Autodesk Fusion 360 part; units mm, degrees
note: some values were not read from the file. Chosen so that the rebuilt part matches the saved one: which face or edge a step refers to. Set by a fixed rule: which sketch regions a step uses.
(part 2 of 2)
sketch "Sketch18" plane through (0, 5, 0) normal (0, 1, 0) x (-1, 0, 0)
  line L0 (114.8227, 27.0674) -> (114.8227, -2.7993)
  line L1 (114.8227, -2.7993) -> (107.5823, -2.7993)
  line L2 (107.5823, -2.7993) -> (107.5823, 27.0674)
  line L3 (107.5823, 27.0674) -> (114.8227, 27.0674)
  line L4 (58, -24) -> (58, -27)
  line L5 (58, -27) -> (18, -27)
  line L6 (18, -27) -> (18, -24)
  line L7 (18, -24) -> (58, -24)
  line L8 (-10.8736, -33.1025) -> (-10.8736, -37.1025)
  line L9 (-10.8736, -37.1025) -> (-40.8736, -37.1025)
  line L10 (-40.8736, -37.1025) -> (-40.8736, -33.1025)
  line L11 (-40.8736, -33.1025) -> (-10.8736, -33.1025)
  circle A0 centre (-6.976, 41.8165) radius 1.5
  line L12 (-78.4638, 67.7606) -> (-78.4638, 30)
  line L13 (-78.4638, 30) -> (-84.4638, 30)
  line L14 (-84.4638, 30) -> (-84.4638, 67.7606)
  line L15 (-84.4638, 67.7606) -> (-78.4638, 67.7606)
  line L16 (-45, 85) -> (-45, 75)
  line L17 (-45, 75) -> (-85, 75)
  line L18 (-85, 75) -> (-85, 85)
  line L19 (-85, 85) -> (-45, 85)
  line L20 (-4.2145, 80) -> (-4.2145, 53.7294)
  line L21 (-4.2145, 53.7294) -> (-9.1198, 53.7294)
  line L22 (-9.1198, 53.7294) -> (-9.1198, 80)
  line L23 (-9.1198, 80) -> (-4.2145, 80)
  line L24 (-82.9645, 18.0619) -> (-82.9645, -13.0755)
  line L25 (-82.9645, -13.0755) -> (-89.1235, -13.0755)
  line L26 (-89.1235, -13.0755) -> (-89.1235, 18.0619)
  line L27 (-89.1235, 18.0619) -> (-82.9645, 18.0619)
  line L28 (44.7011, 105) -> (44.7011, 92.7786)
  line L29 (44.7011, 92.7786) -> (10, 92.7786)
  line L30 (10, 92.7786) -> (10, 105)
  line L31 (10, 105) -> (44.7011, 105)
  line L32 (-100, 38.7801) -> (-100, -17.7685)
  line L33 (-100, -17.7685) -> (-109.4869, -17.7685)
  line L34 (-109.4869, -17.7685) -> (-109.4869, 38.7801)
  line L35 (-109.4869, 38.7801) -> (-100, 38.7801)
  line L36 (0, 105) -> (0, 92.7786)
  line L37 (0, 92.7786) -> (-35, 92.7786)
  line L38 (-35, 92.7786) -> (-35, 105)
  line L39 (-35, 105) -> (0, 105)
  line L40 (-2.8969, 25.8787) -> (-2.8969, -24.0249)
  line L41 (-2.8969, -24.0249) -> (-8.0295, -24.0249)
  line L42 (-8.0295, -24.0249) -> (-8.0295, 25.8787)
  line L43 (-8.0295, 25.8787) -> (-2.8969, 25.8787)
  circle A1 centre (-97.7344, 53.0689) radius 5.2675
  circle A2 centre (97.7344, 53.0689) radius 5.2675
  circle A3 centre (92.5, -14.3) radius 1.6
  circle A4 centre (2.5, 75.7) radius 1.6
  circle A5 centre (92.5, 75.7) radius 1.6
  circle A6 centre (92.5, -17.7) radius 1.6
  circle A7 centre (92.5, -10.9) radius 1.6
  circle A8 centre (2.5, 72.3) radius 1.6
  circle A9 centre (92.5, 72.3) radius 1.6
  circle A10 centre (2.5, -14.3) radius 1.6
  circle A11 centre (-90.9905, 60.7002) radius 1.5
  circle A12 centre (90.8662, 44.7011) radius 1.5
  circle A13 centre (-90.8662, 44.7011) radius 1.5
  circle A14 centre (104.8647, 60.7002) radius 1.5
  circle A15 centre (90.9999, 67.3221) radius 1.5
  circle A16 centre (-104.8647, 60.7002) radius 1.5
  circle A17 centre (105.0292, 44.701) radius 1.5
  arc A18 (-105.0048, 43.2011) -> (-105.0133, 46.2009) centre (-104.989, 44.7011) ccw
  arc A19 (-105.0133, 46.2009) -> (-105.0048, 43.2011) centre (-105.0292, 44.701) ccw
  circle A20 centre (90.8944, 60.7176) radius 1.5
  circle A21 centre (0, -58) radius 2.45
  circle A22 centre (0, -116) radius 2.45
  circle A23 centre (104.95, 64) radius 1.5
  circle A24 centre (-90.95, 48) radius 1.5
  circle A25 centre (104.95, 48) radius 1.5
  circle A26 centre (-90.95, 64) radius 1.5
  circle A27 centre (-104.95, 64) radius 1.5
  circle A28 centre (90.95, 48) radius 1.5
  circle A29 centre (90.95, 64) radius 1.5
  circle A30 centre (-104.95, 48) radius 1.5
  line L44 (74, 33) -> (74, 28)
  line L45 (74, 28) -> (30, 28)
  line L46 (30, 28) -> (30, 33)
  line L47 (30, 33) -> (74, 33)
  line L48 (-30, 28) -> (-74, 28)
  line L49 (-74, 28) -> (-74, 33)
  line L50 (-74, 33) -> (-30, 33)
  line L51 (-30, 33) -> (-30, 28)
  line L52 (-112.5, 43.0811) -> (-117.3415, 43.0811)
  arc A31 (-117.3415, 43.0811) -> (117.3415, 43.0811) centre (0, 0) ccw
  line L53 (117.3415, 43.0811) -> (112.5, 43.0811)
  line L54 (112.5, 43.0811) -> (112.5, 68.0811)
  line L55 (112.5, 68.0811) -> (104.833, 68.0811)
  arc A32 (104.833, 68.0811) -> (-104.833, 68.0811) centre (0, 0) ccw
  line L56 (-104.833, 68.0811) -> (-112.5, 68.0811)
  line L57 (-112.5, 68.0811) -> (-112.5, 43.0811)
  circle A33 centre (91.5428, 79.2656) radius 1.6
  circle A34 centre (2.5, 79.1) radius 1.6
  circle A35 centre (-80.0985, -43.3755) radius 1.7
  circle A36 centre (20.0985, -43.3755) radius 1.7
  circle A37 centre (20.0985, -87.3755) radius 1.7
  circle A38 centre (-20.0985, -87.3755) radius 1.7
  circle A39 centre (-80.0985, -87.3755) radius 1.7
  circle A40 centre (80.0985, -43.3755) radius 1.7
  circle A41 centre (80.0985, -87.3755) radius 1.7
  circle A42 centre (-20.0985, -43.3755) radius 1.7
  line L58 (-85, -25) -> (-65.7302, -25)
  line L59 (-65.7302, -25) -> (-65.7302, -31)
  line L60 (-65.7302, -31) -> (-85, -31)
  line L61 (-85, -31) -> (-85, -25)
  line L62 (102.0125, -33.4763) -> (110, -33.4763)
  line L63 (110, -33.4763) -> (110, -40)
  line L64 (110, -40) -> (102.0125, -40)
  line L65 (102.0125, -40) -> (102.0125, -33.4763)
  dimension "d163" = 6
  constraint horizontal L58
  constraint vertical L59
  constraint horizontal L60
  constraint vertical L61
  constraint horizontal L62
  constraint vertical L63
  constraint horizontal L64
  constraint vertical L65
  measures "d163" distance of L58.start L60.end
extrude "Extrude30" cut sketch "Sketch18" against normal blind 5 contours L58 L59 L60 L61 | L62 L63 L64 L65 bodies 1
sketch "Sketch19" plane through (0, 0, 0) normal (0, -1, 0) x (1, 0, 0)
  circle A0 centre (20.0985, -43.3755) radius 1.7
  circle A1 centre (-80.0985, -87.3755) radius 1.7
  circle A2 centre (-80.0985, -43.3755) radius 1.7
  circle A3 centre (80.0985, -87.3755) radius 1.7
  circle A4 centre (20.0985, -87.3755) radius 1.7
  circle A5 centre (-20.0985, -87.3755) radius 1.7
  circle A6 centre (-20.0985, -43.3755) radius 1.7
  circle A7 centre (80.0985, -43.3755) radius 1.7
  circle A8 centre (-2.5, 79.1) radius 1.6
  circle A9 centre (-91.5428, 79.2656) radius 1.6
  line L0 (117.3415, 43.0811) -> (112.5, 43.0811)
  line L1 (112.5, 43.0811) -> (112.5, 68.0811)
  line L2 (112.5, 68.0811) -> (104.833, 68.0811)
  arc A10 (104.833, 68.0811) -> (-104.833, 68.0811) centre (0, 0) ccw
  line L3 (-104.833, 68.0811) -> (-112.5, 68.0811)
  line L4 (-112.5, 68.0811) -> (-112.5, 43.0811)
  line L5 (-112.5, 43.0811) -> (-117.3415, 43.0811)
  arc A11 (-117.3415, 43.0811) -> (-10, -124.5994) centre (0, 0) ccw
  line L6 (-10, -124.5994) -> (-10, -45)
  line L7 (-10, -45) -> (10, -45)
  line L8 (10, -45) -> (10, -124.5994)
  arc A12 (10, -124.5994) -> (117.3415, 43.0811) centre (0, 0) ccw
  line L9 (74, 28) -> (30, 28)
  line L10 (30, 28) -> (30, 33)
  line L11 (30, 33) -> (74, 33)
  line L12 (74, 33) -> (74, 28)
  line L13 (-74, 28) -> (-74, 33)
  line L14 (-74, 33) -> (-30, 33)
  line L15 (-30, 33) -> (-30, 28)
  line L16 (-30, 28) -> (-74, 28)
  circle A13 centre (104.95, 48) radius 1.5
  circle A14 centre (-90.95, 64) radius 1.5
  circle A15 centre (-90.95, 48) radius 1.5
  circle A16 centre (104.95, 64) radius 1.5
  circle A17 centre (90.95, 64) radius 1.5
  circle A18 centre (-104.95, 48) radius 1.5
  circle A19 centre (90.95, 48) radius 1.5
  circle A20 centre (-104.95, 64) radius 1.5
  circle A21 centre (-90.8944, 60.7176) radius 1.5
  arc A22 (105.0133, 46.2009) -> (105.0048, 43.2011) centre (104.989, 44.7011) ccw
  arc A23 (105.0048, 43.2011) -> (105.0133, 46.2009) centre (105.0292, 44.701) ccw
  circle A24 centre (-105.0292, 44.701) radius 1.5
  circle A25 centre (-90.9999, 67.3221) radius 1.5
  circle A26 centre (-104.8647, 60.7002) radius 1.5
  circle A27 centre (90.8662, 44.7011) radius 1.5
  circle A28 centre (-90.8662, 44.7011) radius 1.5
  circle A29 centre (-2.5, -14.3) radius 1.6
  circle A30 centre (-92.5, 72.3) radius 1.6
  circle A31 centre (-2.5, 72.3) radius 1.6
  circle A32 centre (-92.5, -10.9) radius 1.6
  circle A33 centre (-92.5, -17.7) radius 1.6
  circle A34 centre (-92.5, 75.7) radius 1.6
  circle A35 centre (-2.5, 75.7) radius 1.6
  circle A36 centre (-92.5, -14.3) radius 1.6
  circle A37 centre (-97.7344, 53.0689) radius 5.2675
  circle A38 centre (97.7344, 53.0689) radius 5.2675
  line L17 (2.8969, -24.0249) -> (2.8969, 25.8787)
  line L18 (2.8969, 25.8787) -> (8.0295, 25.8787)
  line L19 (8.0295, 25.8787) -> (8.0295, -24.0249)
  line L20 (8.0295, -24.0249) -> (2.8969, -24.0249)
  line L21 (0, 92.7786) -> (0, 105)
  line L22 (0, 105) -> (35, 105)
  line L23 (35, 105) -> (35, 92.7786)
  line L24 (35, 92.7786) -> (0, 92.7786)
  line L25 (100, -17.7685) -> (100, 38.7801)
  line L26 (100, 38.7801) -> (109.4869, 38.7801)
  line L27 (109.4869, 38.7801) -> (109.4869, -17.7685)
  line L28 (109.4869, -17.7685) -> (100, -17.7685)
  line L29 (-44.7011, 92.7786) -> (-44.7011, 105)
  line L30 (-44.7011, 105) -> (-10, 105)
  line L31 (-10, 105) -> (-10, 92.7786)
  line L32 (-10, 92.7786) -> (-44.7011, 92.7786)
  line L33 (82.9645, -13.0755) -> (82.9645, 18.0619)
  line L34 (82.9645, 18.0619) -> (89.1235, 18.0619)
  line L35 (89.1235, 18.0619) -> (89.1235, -13.0755)
  line L36 (89.1235, -13.0755) -> (82.9645, -13.0755)
  line L37 (4.2145, 53.7294) -> (4.2145, 80)
  line L38 (4.2145, 80) -> (9.1198, 80)
  line L39 (9.1198, 80) -> (9.1198, 53.7294)
  line L40 (9.1198, 53.7294) -> (4.2145, 53.7294)
  line L41 (45, 75) -> (45, 85)
  line L42 (45, 85) -> (85, 85)
  line L43 (85, 85) -> (85, 75)
  line L44 (85, 75) -> (45, 75)
  line L45 (78.4638, 30) -> (78.4638, 67.7606)
  line L46 (78.4638, 67.7606) -> (84.4638, 67.7606)
  line L47 (84.4638, 67.7606) -> (84.4638, 30)
  line L48 (84.4638, 30) -> (78.4638, 30)
  circle A39 centre (6.976, 41.8165) radius 1.5
  line L49 (-114.8227, -2.7993) -> (-114.8227, 27.0674)
  line L50 (-114.8227, 27.0674) -> (-107.5823, 27.0674)
  line L51 (-107.5823, 27.0674) -> (-107.5823, -2.7993)
  line L52 (-107.5823, -2.7993) -> (-114.8227, -2.7993)
  line L53 (65.7302, -31) -> (65.7302, -25)
  line L54 (65.7302, -25) -> (85, -25)
  line L55 (85, -25) -> (85, -31)
  line L56 (85, -31) -> (65.7302, -31)
  line L57 (-110, -40) -> (-110, -33.4763)
  line L58 (-110, -33.4763) -> (-102.0125, -33.4763)
  line L59 (-102.0125, -33.4763) -> (-102.0125, -40)
  line L60 (-102.0125, -40) -> (-110, -40)
  arc A40 (17, -122) -> (74.3564, -98.5123) centre (0.1514, 0.9191) ccw
  line L61 (0, -124) -> (0, -59) construction
  line L62 (74.3564, -98.5123) -> (75.9114, -99.3099)
  line L63 (17, -122) -> (17, -123.8386)
  arc A41 (90.5, -84.5) -> (122.1341, -18.16) centre (-0.7621, -0.2695) ccw
  line L64 (122.1341, -18.16) -> (123.6738, -18.16)
  line L65 (90.5, -84.5) -> (91.4094, -85.2603)
  arc A42 (76.2789, 96.4429) -> (6.6664, 123.005) centre (2.8431, 8.486) ccw
  line L66 (76.2789, 96.4429) -> (77.7474, 97.8792)
  line L67 (6.6664, 123.005) -> (6.6664, 124.8221)
  arc A43 (-6.6664, 123.005) -> (-76.2789, 96.4429) centre (-2.8431, 8.486) ccw
  line L68 (-76.2789, 96.4429) -> (-77.7474, 97.8792)
  line L69 (-6.6664, 123.005) -> (-6.6664, 124.8221)
  line L70 (-122.1341, -18.16) -> (-123.6738, -18.16)
  arc A44 (-122.1341, -18.16) -> (-90.5, -84.5) centre (0.7621, -0.2695) ccw
  line L71 (-90.5, -84.5) -> (-91.4094, -85.2603)
  line L72 (-74.3564, -98.5123) -> (-75.9114, -99.3099)
  arc A45 (-74.3564, -98.5123) -> (-17, -122) centre (-0.1514, 0.9191) ccw
  line L73 (-17, -122) -> (-17, -123.8386)
  line L74 (55, -105) -> (35, -105)
  line L75 (35, -105) -> (35, -100)
  line L76 (35, -100) -> (55, -100)
  line L77 (55, -100) -> (55, -105)
  line L78 (-55, -100) -> (-55, -105)
  line L79 (-55, -105) -> (-35, -105)
  line L80 (-35, -100) -> (-55, -100)
  line L81 (-35, -105) -> (-35, -100)
  circle A46 centre (104.8647, 60.7002) radius 1.5
  circle A47 centre (90.9905, 60.7002) radius 1.5
  constraint tangent A12 A40
  constraint vertical L61
  constraint coincident A12 L62.end
  constraint coincident A12 L63.end
  constraint vertical L63
  constraint tangent A12 A41
  constraint coincident A12 L64.end
  constraint horizontal L64
  constraint coincident A12 L65.end
  constraint coincident A10 L66.end
  constraint coincident A10 L67.end
  constraint vertical L67
  constraint symmetric A40.end L61 L72.start
  constraint symmetric A40.start L61 A45.end
  constraint symmetric A40 L61 A45
  constraint symmetric L61 L62.end L72.end
  constraint symmetric L61 L63.end L73.end
  constraint symmetric L61 A41.start A44.end
  constraint symmetric L61 A41.end L70.start
  constraint symmetric L61 A41 A44
  constraint symmetric L61 L64.end L70.end
  constraint symmetric L61 L65.end L71.end
  constraint symmetric L61 A42.start A43.end
  constraint symmetric L61 A42.end A43.start
  constraint symmetric L61 A42 A43
  constraint symmetric L61 L66.end L68.end
  constraint symmetric L61 L67.end L69.end
  constraint horizontal L74
  constraint vertical L75
  constraint horizontal L76
  constraint vertical L77
  constraint symmetric L61 L74.start L78.end
  constraint symmetric L61 L74.end L79.end
  constraint symmetric L61 L75.end L80.start
  constraint symmetric L61 L76.end L78.start
extrude "Extrude31" add sketch "Sketch19" along normal blind 7 contours A12 A41 L64 L65 | A12 A40 L62 L63 | A10 A42 L66 L67 | A10 A43 L68 L69 | A11 L72 A45 L73 | A11 L70 A44 L71 bodies 1
sketch "Sketch20" plane through (0, -7, 0) normal (0, -1, 0) x (1, 0, 0)
  line L0 (76.2789, 96.4429) -> (77.7474, 97.8792)
  arc A0 (77.7474, 97.8792) -> (6.6664, 124.8221) centre (0, 0) ccw
  line L1 (6.6664, 124.8221) -> (6.6664, 123.005)
  arc A1 (76.2789, 96.4429) -> (6.6664, 123.005) centre (2.8431, 8.486) ccw
  arc A2 (-6.6664, 123.005) -> (-76.2789, 96.4429) centre (-2.8431, 8.486) ccw
  line L2 (-6.6664, 123.005) -> (-6.6664, 124.8221)
  arc A3 (-6.6664, 124.8221) -> (-77.7474, 97.8792) centre (0, 0) ccw
  line L3 (-77.7474, 97.8792) -> (-76.2789, 96.4429)
  arc A4 (76.2789, 96.4429) -> (6.6664, 123.005) centre (2.8431, 8.486) ccw
  arc A5 (76.3242, 96.4971) -> (6.6688, 123.0757) centre (2.8431, 8.486) ccw
  arc A6 (75.4269, 95.4225) -> (6.6221, 121.6765) centre (2.8431, 8.486) ccw
  line L4 (6.6221, 121.6765) -> (6.6664, 123.005)
  line L5 (75.4269, 95.4225) -> (76.2789, 96.4429)
  arc A7 (-6.6197, 121.6058) -> (-75.3816, 95.3682) centre (-2.8431, 8.486) ccw
  line L6 (-6.6197, 121.6058) -> (-6.6664, 123.005)
  line L7 (-75.3816, 95.3682) -> (-76.2789, 96.4429)
  arc A8 (90.5, -84.5) -> (122.1341, -18.16) centre (-0.7621, -0.2695) ccw
  line L8 (90.5, -84.5) -> (91.4094, -85.2603)
  arc A9 (91.4094, -85.2603) -> (123.6738, -18.16) centre (0, 0) ccw
  line L9 (123.6738, -18.16) -> (122.1341, -18.16)
  arc A10 (17, -122) -> (74.3564, -98.5123) centre (0.1514, 0.9191) ccw
  line L10 (17, -122) -> (17, -123.8386)
  arc A11 (17, -123.8386) -> (75.9114, -99.3099) centre (0, 0) ccw
  line L11 (75.9114, -99.3099) -> (74.3564, -98.5123)
  arc A12 (16.8099, -120.613) -> (73.5191, -97.3903) centre (0.1514, 0.9191) ccw
  arc A13 (89.4712, -83.5505) -> (120.7487, -17.9583) centre (-0.7621, -0.2695) ccw
  line L12 (89.4712, -83.5505) -> (90.5, -84.5)
  line L13 (120.7487, -17.9583) -> (122.1341, -18.16)
  line L14 (73.5191, -97.3903) -> (74.3564, -98.5123)
  line L15 (16.8099, -120.613) -> (17, -122)
  line L16 (0, -126) -> (0, -45) construction
  line L17 (0, -126) -> (0, -45) construction
  arc A14 (-73.5191, -97.3903) -> (-16.8099, -120.613) centre (-0.1514, 0.9191) ccw
  line L18 (-16.8099, -120.613) -> (-17, -122)
  line L19 (-73.5191, -97.3903) -> (-74.3564, -98.5123)
  line L20 (-89.4712, -83.5505) -> (-90.5, -84.5)
  arc A15 (-120.7487, -17.9583) -> (-89.4712, -83.5505) centre (0.7621, -0.2695) ccw
  line L21 (-120.7487, -17.9583) -> (-122.1341, -18.16)
  line L22 (-74.3564, -98.5123) -> (-75.9114, -99.3099)
  arc A16 (-75.9114, -99.3099) -> (-17, -123.8386) centre (0, 0) ccw
  line L23 (-17, -123.8386) -> (-17, -122)
  arc A17 (-74.3564, -98.5123) -> (-17, -122) centre (-0.1514, 0.9191) ccw
  line L24 (-122.1341, -18.16) -> (-123.6738, -18.16)
  arc A18 (-123.6738, -18.16) -> (-91.4094, -85.2603) centre (0, 0) ccw
  line L25 (-91.4094, -85.2603) -> (-90.5, -84.5)
  arc A19 (-122.1341, -18.16) -> (-90.5, -84.5) centre (0.7621, -0.2695) ccw
  dimension "d168" = -1.4
  dimension "d169" = -1.4
  dimension "d172" = -1.4
  dimension "d173" = -1.4
  constraint coincident A2.start L2.start
  constraint coincident A2.end L3.end
  constraint coincident A8.start L8.start
  constraint coincident A8.end L9.end
  constraint coincident A10.end L11.end
  constraint coincident A10.start L10.start
  constraint vertical L16
  constraint symmetric A12.end L16 A14.start
  constraint symmetric A12.start L16 A14.end
  constraint symmetric A12 L16 A14
  constraint symmetric A13.end L16 A15.start
  constraint symmetric A13.start L16 L20.start
  constraint symmetric A13 L16 A15
  constraint symmetric A8.start L16 L20.end
  constraint symmetric A8.end L16 L21.end
  constraint symmetric A10.end L16 L19.end
  constraint symmetric A10.start L16 L18.end
  constraint symmetric L17.start L16 L16.start
  constraint symmetric L17.end L16 L16.end
extrude "Extrude32" add sketch "Sketch20" along normal blind 2 separate body contours A1 A4 A6 L4 L5 | A2 A7 L6 L7 | A8 A13 L12 L13 | A10 A12 L14 L15 | A14 L18 L19 A17 | L20 A15 L21 A19 makes body 2 at (72.325, -7.6667, 99.5985) makes body 3 at (-31.6505, -8.3333, 119.3885) makes body 4 at (93.7996, -7.6667, -80.7781) makes body 5 at (27.2719, -8.3333, -120.1489) makes body 6 at (-70.1084, -7.6667, -101.5456) makes body 7 at (-105.4319, -7.6667, -64.6619)
